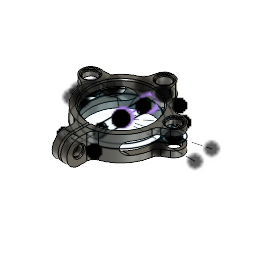
hw4 (Autodesk Fusion 360 design; units mm, degrees)
part number: 2026-08-06-14-05-16-877
Autodesk Fusion 360 part; units mm, degrees
sketch "스케치1" plane through (0, 0, 0) normal (0, 0, 1) x (1, 0, 0)
  circle A0 centre (0, 0) radius 25
  circle A1 centre (0, 0) radius 30
  circle A2 centre (0, 35) radius 5
  circle A3 centre (0, 35) radius 7.5
  line L0 (0, 0) -> (0, 35) construction
  line L1 (7.2444, 36.9411) -> (8.7332, 31.3852)
  arc A4 (8.7332, 31.3852) -> (12.1073, 27.4484) centre (14.5287, 32.9381) ccw
  line L2 (0, 0) -> (57.9555, 15.5291) construction
  line L3 (0, 0) -> (60, 0) construction
  circle A5 centre (33.8074, 9.0587) radius 5
  circle A6 centre (33.8074, 9.0587) radius 7.5
  line L4 (33.8074, 16.5587) -> (25.0162, 16.5587)
  line L5 (37.5574, 2.5635) -> (29.944, -1.8321)
  line L6 (14.5287, 32.9381) -> (0, 0) construction
  line L7 (28.0554, 22.5587) -> (0, 0) construction
  arc A7 (23.3795, 18.7989) -> (28.0554, 16.5587) centre (28.0554, 22.5587) ccw
  arc A8 (33.1981, 0) -> (29.6467, -4.5906) centre (35.576, -5.5087) ccw
  line L8 (-14.5287, 32.9381) -> (0, 0) construction
  line L9 (-33.8074, 16.5587) -> (-25.0162, 16.5587)
  line L10 (-37.5574, 2.5635) -> (-29.944, -1.8321)
  circle A9 centre (-33.8074, 9.0587) radius 7.5
  arc A10 (-12.1073, 27.4484) -> (-8.7332, 31.3852) centre (-14.5287, 32.9381) ccw
  line L11 (-28.0554, 22.5587) -> (0, 0) construction
  line L12 (0, 0) -> (0, 35) construction
  arc A11 (-29.6467, -4.5906) -> (-33.1981, 0) centre (-35.576, -5.5087) ccw
  line L13 (-7.2444, 36.9411) -> (-8.7332, 31.3852)
  arc A12 (-28.0554, 16.5587) -> (-23.3795, 18.7989) centre (-28.0554, 22.5587) ccw
  circle A13 centre (-33.8074, 9.0587) radius 5
  arc A14 (-6, -33.9411) -> (-10, -28.2843) centre (-12, -33.9411) ccw
  arc A15 (10, -28.2843) -> (6, -33.9411) centre (12, -33.9411) ccw
  line L14 (-6, -33.9411) -> (6, -33.9411)
  line L15 (0, 0) -> (0, -33.9411) construction
  line L16 (0, -33.9411) -> (-12, -33.9411) construction
  line L17 (0, -33.9411) -> (12, -33.9411) construction
  point P0 (0, 35)
  point P1 (0, 35)
  dimension "d1" = 50
  dimension "d2" = 60
  dimension "d3" = 10
  dimension "d5" = 35
  dimension "d6" = 15
  dimension "d7" = 12
  dimension "d9" = 15
  dimension "d10" = 60
  dimension "d11" = 60
  dimension "d12" = 15
  dimension "d13" = 10
  dimension "d14" = 15
  dimension "d15" = 35
  dimension "d19" = 30
  dimension "d20" = 12
  dimension "d21" = 12
  dimension "d23" = 27.396
  dimension "d41" = 6
  dimension "d42" = 33.9411
  dimension "d43" = 12
  constraint coincident A0.centre A1.centre
  constraint concentric A2 A3
  constraint vertical L0
  constraint coincident P1 L0
  constraint tangent A3 L1
  constraint tangent L1 A4
  constraint tangent A1 A4
  constraint coincident A3 L1.start
  constraint coincident P1 P0
  constraint coincident A1 A4.end
  constraint perpendicular L0 L3
  constraint coincident L2 A5.centre
  constraint concentric A5 A6
  constraint tangent A6 L4
  constraint tangent A1 A7
  constraint tangent L4 A7
  constraint tangent A6 L5
  constraint coincident A1 L4.end
  constraint coincident A1 L5.end
  constraint tangent L5 A8
  constraint tangent A1 A8
  constraint coincident A6 L5.start
  constraint coincident A6 L4.start
  constraint coincident A4.centre L6.start
  constraint coincident L7.start A7.centre
  constraint coincident L4 A7.end
  constraint coincident A1 A7.start
  constraint coincident A1 A8.end
  constraint coincident L3 A8.start
  constraint symmetric A0.centre L0 A1.centre
  constraint symmetric P1 L0 P0
  constraint symmetric L0 L1.end A10.end
  constraint symmetric L0 L1.start L13.start
  constraint symmetric L0 A4.end A10.start
  constraint symmetric L0 A4 A10
  constraint symmetric L0 A0.centre A1.centre
  constraint symmetric L0 A5 A13
  constraint symmetric L0 A6 A9
  constraint symmetric L0 L4.end L9.end
  constraint symmetric L0 L5.end L10.end
  constraint symmetric L0 L5.start L10.start
  constraint symmetric L0 L4.start L9.start
  constraint symmetric L0 A4.centre L8.start
  constraint symmetric L0 L7.start L11.start
  constraint symmetric L0 A7.end A12.start
  constraint symmetric L0 A7.start A12.end
  constraint symmetric L0 A7 A12
  constraint symmetric L0 A8.end A11.start
  constraint symmetric L0 A8 A11
  constraint symmetric L0 A8.start A11.end
  constraint coincident L11.start A12.centre
  constraint tangent A1 A15
  constraint coincident A1 A14.end
  constraint coincident A1 A15.start
  constraint midpoint L14 L15.end
  constraint vertical L15
  constraint perpendicular L15 L16
  constraint coincident A14.centre L16.end
  constraint coincident A15.centre L17.end
  constraint perpendicular L15 L17
  measures "d1" diameter of A0
  measures "d2" diameter of A1
  measures "d3" diameter of A2
  measures "d5" distance of A0.centre P1
  measures "d6" diameter of A3
  measures "d7" diameter of A4
  measures "d9" angle of L0 L1
  measures "d10" distance of A0.centre L2.end
  measures "d11" distance of A0.centre L3.end
  measures "d12" angle of L2 L3
  measures "d13" diameter of A5
  measures "d14" diameter of A6
  measures "d15" distance of A0.centre A5.centre
  measures "d19" angle of L4 L5
  measures "d20" diameter of A7
  measures "d21" diameter of A8
  measures "d23" angle of L6 L7
  measures "d41" radius of A14
  measures "d42" distance of L3 L14
  measures "d43" distance of A15.end A14.start
extrude "돌출1" add sketch "스케치1" along normal mid plane 20 contours A1 A3 A6 A9 | A1 A6 L4 | A1 L4 A7 | A1 A6 | A1 A6 | A1 A3 L1 A4 | A1 A6 L5 | A1 A3 | A1 A3 | A1 A3 A10 L13 | A1 L5 A8 | A1 L9 A9 | A1 A9 | A1 A9 | A1 L10 A9 makes body 1
sketch "스케치3" plane through (0, 0, 0) normal (1, 0, 0) x (0, 1, 0)
  line L0 (0, 0) -> (-40, 0) construction
  circle A0 centre (-17, 0) radius 5
  circle A1 centre (18, 0) radius 5
  line L1 (1.75, 0) -> (22.5, 0)
  line L2 (18, 5) -> (-17, 5)
  line L3 (18, -5) -> (-17, -5)
  dimension "d29" = 40
  dimension "d30" = 10
  dimension "d31" = 23
  dimension "d32" = 10
  dimension "d33" = 35
  constraint coincident L0.start origin
  constraint horizontal L0
  constraint coincident L0 A0.centre
  constraint coincident A1.centre L1
  constraint coincident A1 L2.start
  constraint coincident A0 L2.end
  constraint parallel L0 L2
  constraint tangent A0 L2
  constraint horizontal L3
  constraint tangent A0 L3
  constraint coincident A0 L3.end
  constraint coincident A1 L3.start
  measures "d29" distance of L0.start L0.end
  measures "d30" diameter of A0
  measures "d31" horizontal distance of L0.end A0.centre
  measures "d32" diameter of A1
  measures "d33" horizontal distance of A0.centre A1.centre
extrude "돌출2" cut sketch "스케치3" along normal mid plane 200 bodies 1
extrude "돌출3" add sketch "스케치1" along normal mid plane 20 separate body contours A1 A14 A15 L14 makes body 2
sketch "스케치6" plane through (0, 0, 0) normal (1, 0, 0) x (0, 1, 0)
  circle A0 centre (-40, 0) radius 4
  line L0 (0, 0) -> (-50, 0) construction
  circle A1 centre (-40, 0) radius 10
  line L1 (-33.9411, -10) -> (-33.9411, 10)
  line L2 (-33.9411, -10) -> (-40, -10)
  line L3 (-33.9411, 10) -> (-40, 10)
  point P0 (-17, 0)
  point P1 (-33.9411, 0)
  dimension "d46" = 8
  dimension "d47" = 23
  dimension "d49" = 20
  dimension "d50" = 20
  constraint coincident L0.start origin
  constraint horizontal L0
  constraint coincident A0.centre L0
  constraint concentric A0 A1
  constraint perpendicular L0 L1
  constraint perpendicular L1 L2
  constraint tangent A1 L2
  constraint perpendicular L1 L3
  constraint coincident L1 P1
  constraint coincident A1 L3.end
  constraint coincident A1 L2.end
  constraint coincident L0.end A1
  measures "d46" diameter of A0
  measures "d47" horizontal distance of A0.centre P0
  measures "d49" diameter of A1
  measures "d50" distance of L1.start L1.end
extrude "돌출4" add sketch "스케치6" along normal mid plane 12 contours A1 L1 | A1 L1 L3 | A1 L1 L2 picked at (-34.6274, 0) bodies 2
sketch "스케치7" plane through (0, 0, 0) normal (0, 0, 1) x (1, 0, 0)
  line L0 (-1, -20) -> (1, -20)
  line L1 (1, -20) -> (1, -50)
  line L2 (1, -50) -> (-1, -50)
  line L3 (-1, -50) -> (-1, -20)
  point P0 (0, -40)
  dimension "d53" = 2
  dimension "d54" = 30
  dimension "d55" = 1
  dimension "d56" = 20
  constraint horizontal L0
  constraint vertical L1
  constraint horizontal L2
  constraint vertical L3
  measures "d53" distance of L0.start L0.end
  measures "d54" distance of L0.start L2.end
  measures "d55" horizontal distance of L1.end P0
  measures "d56" vertical distance of L0.end origin
extrude "돌출5" cut sketch "스케치7" along normal mid plane 20 bodies 1 2 makes body 3 at (-1, -31.9889, 0)
chamfer "챔퍼1" distance 1 angle 45 5 edges at (6, -43.7293, 1.4465) (0, 25, 10) (-38.469, 10.8667, 10) (-4.6616, 36.8081, 10) (29.1458, 10.8667, 10) on bodies 1 2
chamfer "챔퍼2" distance 1 angle 45 4 edges at (-6, -43.7293, -1.4465) (-38.469, 7.2506, -10) (-4.6616, 33.1919, -10) (29.1458, 7.2506, -10) on bodies 1 3
fillet "필렛1" radius 1 1 edges at (-39.4014, 11.2284, -10) on bodies 1
fillet "필렛2" radius 1 6 edges at (-38.469, 7.2506, -9) (-4.6616, 33.1919, -9) (-5.594, 37.1697, -10) (28.2134, 11.2284, -10) (29.1458, 7.2506, -9) (5, -43.7293, 1.4465) on bodies 1 2
fillet "필렛3" radius 1 8 edges at (29.1458, 10.8667, 9) (28.2134, 6.889, 10) (-5.594, 32.8303, 10) (-4.6616, 36.8081, 9) (-39.4014, 6.889, 10) (-38.469, 10.8667, 9) (-6, -44.6616, 1.8081) (-5, -43.7293, -1.4465) on bodies 1 3
